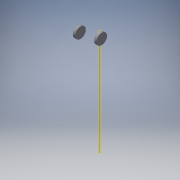
# Autodesk Inventor part: rodamientos medio
Saved by Autodesk Inventor 2016 (Build 200138000, 138)
## iProperties
Created: 2016-07-27
Part Number: rodamientos medio
Material: Generic
Document SubType Name: Modeling
Designer: Admin
Density: 1 g/cm^3
Appearance: Default
Author: Admin
Autodesk Inventor part; units mm, degrees
ref_plane "YZ Plane" through (0, 0, 0) normal (1, 0, 0) x (0, 1, 0)
ref_plane "XZ Plane" through (0, 0, 0) normal (0, 1, 0) x (-1, 0, 0)
ref_plane "XY Plane" through (0, 0, 0) normal (0, 0, 1) x (1, 0, 0)
ref_plane "Work Plane1" through (-263.7089, -187.9059, -236.5724) normal (1, 0, 0) x (0, 1, 0)
sketch "Sketch1" plane through (-263.7089, -187.9059, -236.5724) normal (1, 0, 0) x (0, 1, 0)
  circle A0 centre (-6, -6) radius 25
  point P0 (187.9059, 236.5724)
  dimension "d0" = 50
  constraints: 1 centre point
  measures "d0" diameter of A0
extrude "Extrusion1" add sketch "Sketch1" along normal blind 10
sketch "Sketch3" plane through (-253.7089, -193.9059, -242.5724) normal (1, 0, 0) x (0, 0, -1)
  circle A0 centre (0, 0) radius 2.25
  point P0 (-242.5724, 193.9059)
  dimension "d7" = 4.5
  constraints: 1 centre point
  measures "d7" diameter of A0
extrude "Extrusion3" cut sketch "Sketch3" against normal blind 10
body "Solid1"
